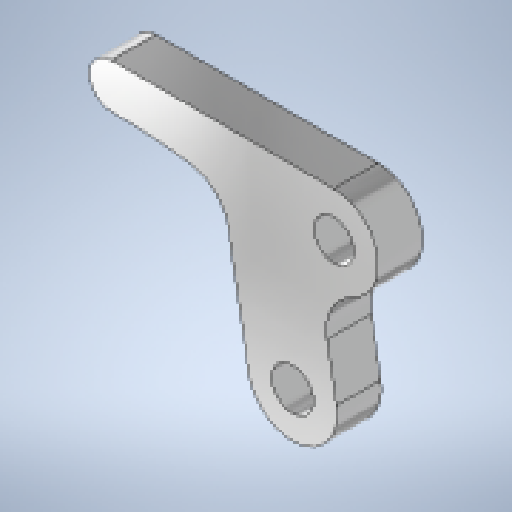
# Autodesk Inventor part: Lever
Saved by Autodesk Inventor 2023.4 (Build 274418000, 418)
## iProperties
Created: 2024-02-17
Part Number: Lever
Material: Aluminum 6061
Document SubType Name: Modeling
Designer: Nathan Cai
Density: 2.7 g/cm^3
Appearance: Aluminum - Flat
Author: Nathan Cai
Autodesk Inventor part; units mm, degrees
ref_plane "YZ Plane" through (0, 0, 0) normal (1, 0, 0) x (0, 1, 0)
ref_plane "XZ Plane" through (0, 0, 0) normal (0, 1, 0) x (-1, 0, 0)
ref_plane "XY Plane" through (0, 0, 0) normal (0, 0, 1) x (1, 0, 0)
sketch "Sketch1" plane through (0, 0, 0) normal (0, 0, 1) x (1, 0, 0)
  circle A0 centre (0, 0) radius 1.4224
  circle A1 centre (0, 0) radius 3.175
  line L0 (0, 0) -> (-19.05, 0) construction
  circle A2 centre (-2.9467, -10.7147) radius 3.175
  circle A3 centre (-2.9467, -10.7147) radius 5 construction
  circle A4 centre (-2.9467, -10.7147) radius 1.5
  line L1 (0, 0) -> (-2.9467, -10.7147) construction
  line L2 (-2.9467, -10.7147) -> (-4.393, -10.3169) construction
  line L3 (0, 0) -> (-2.9467, -10.7147) construction
  arc A5 (-6.0135, -9.8929) -> (0.1201, -11.5364) centre (-2.9467, -10.7147) ccw
  arc A6 (-1.0297, -3.0034) -> (-19.05, 0) centre (-19.05, -55.5625) ccw
  arc A7 (-19.05, 3.175) -> (-19.05, 0) centre (-19.05, 1.5875) ccw
  line L4 (-19.05, 3.175) -> (0, 3.175)
  line L5 (-2.9467, -10.7147) -> (-4.836, 0) construction
  line L6 (0.1801, -10.1634) -> (-1.7092, 0.5513)
  line L7 (-7.9627, -0.5513) -> (-6.0734, -11.266)
  arc A8 (-6.0734, -11.266) -> (0.1801, -10.1634) centre (-2.9467, -10.7147) ccw
  arc A9 (-1.7092, 0.5513) -> (-7.9627, -0.5513) centre (-4.836, 0) ccw
  circle A10 centre (6.7469, -0.7937) radius 3.175
  circle A11 centre (6.7469, -0.7937) radius 1.5
  line L8 (7.1178, 2.3595) -> (0.371, 3.1533)
  arc A12 (4.769, -3.2774) -> (-0.4834, -6.4004) centre (2.7339, -5.8331) ccw
  circle A13 centre (6.7469, -0.7937) radius 5 construction
  point P0 (0.1201, -11.5364)
  point P1 (0, 3.175)
  point P2 (-7.8592, -1.1386)
  point P3 (-6.0734, -11.266)
  point P4 (0.1801, -10.1634)
  point P5 (-1.0859, -2.9835)
  point P6 (-2.418, 2.0577)
  point P7 (0.6312, -3.1116)
  point P8 (1.3474, -2.8749)
  point P9 (-1.4243, -1.0642)
  point P10 (-1.7024, 0.5129)
  point P11 (0.1801, -10.1634)
  dimension "d24" = 3
  dimension "d0" = 2.8448
  dimension "d1" = 6.35
  dimension "d9" = 19.05
  dimension "d22" = 6.35
  dimension "d23" = 10
  dimension "d26" = 11.1125
  dimension "d29" = 3.175
  dimension "d30" = 6.35
  dimension "d31" = 6.35
  dimension "d32" = 3
  dimension "d36" = 10
  dimension "d37" = 100
  dimension "d38" = 4.7625
  dimension "d39" = 6.7469
  dimension "d40" = 0.7937
  constraints: 22 end point, 17 point on circle, 14 tangent, 13 centre point, 6 coincident, 2 point on line, 1 concentric, 1 horizontal, 1 parallel, 1 perpendicular, 3 other
  measures "d0" diameter of A0
  measures "d1" diameter of A1
  measures "d9" distance of L0.start L0.end
  measures "d22" diameter of A2
  measures "d23" diameter of A3
  measures "d26" distance from line of point (0, 0) L2
  measures "d29" diameter of A7
  measures "d30" diameter of A9
  measures "d31" diameter of A10
  measures "d32" diameter of A11
  measures "d36" diameter of A13
  measures "d37" angle of L0 L5
  measures "d38" distance from line of A0.centre L5
  measures "d39" horizontal distance of A0.centre A11.centre
  measures "d40" vertical distance of A0.centre A11.centre
extrude "Extrusion1" add sketch "Sketch1" along normal blind 3.175 contours A1 L6 A9 | A12 L6 A1 | A1 A9 L4 | L6 A2 L7 A6 | A9 L6 A1 | A1 A6 L7 A9 | A9 L7 A6 A7 L4 | A2
fillet "Fillet1" radius 3.175 1 edges at (-7.8592, -1.1386, 1.5875)
sketch "Sketch2" plane through (0, 0, 3.175) normal (0, 0, 1) x (1, 0, 0)
  circle A0 centre (-2.9467, -10.7147) radius 1.5 projected
  circle A1 centre (-2.9467, -10.7147) radius 5.5
  line L0 (0, 3.175) -> (-19.05, 3.175) projected
  arc A2 (-19.05, 3.175) -> (-19.05, 0) centre (-19.05, 1.5875) ccw projected
  arc A3 (-10.0913, -0.727) -> (-19.05, 0) centre (-19.05, -55.5625) ccw projected
  arc A4 (-7.4765, -3.3091) -> (-10.0913, -0.727) centre (-10.6032, -3.8604) ccw projected
  line L1 (-7.4765, -3.3091) -> (-6.0734, -11.266) projected
  arc A5 (-6.0734, -11.266) -> (0.1801, -10.1634) centre (-2.9467, -10.7147) ccw projected
  line L2 (0.1801, -10.1634) -> (-0.4834, -6.4004) projected
  arc A6 (1.3474, -2.8749) -> (-0.4834, -6.4004) centre (2.7339, -5.8331) ccw projected
  arc A7 (1.3474, -2.8749) -> (0, 3.175) centre (0, 0) ccw projected
  circle A8 centre (0, 0) radius 1.4224 projected
  circle A9 centre (-2.9467, -10.7147) radius 1.5 projected
  arc A10 (-7.4765, -3.3091) -> (-10.0913, -0.727) centre (-10.6032, -3.8604) ccw projected
  line L3 (0, 3.175) -> (-19.05, 3.175) projected
  arc A11 (-7.4765, -3.3091) -> (-5.6965, 3.175) centre (-18.3965, 3.175) ccw
  point P0 (-6.8533, -6.8432)
  point P1 (-0.5325, -5.7729)
  point P2 (-5.6965, 3.175)
  dimension "d41" = 11
  dimension "d42" = 12.7
  constraints: 2 centre point, 2 point on circle, 1 coincident, 1 line through centre, 1 point on line
  measures "d41" diameter of A1
  measures "d42" radius of A11
extrude "Extrusion2" add sketch "Sketch2" along normal blind 0.7937 contours A1 L1 A11 L0 A7 A6 | A4 A3 A2 L0 A11
extrude "Extrusion3" add sketch "Sketch2" along normal blind 3.175 contours A1 L1 A11 L0 A7 A6
fillet "Fillet2" radius 1.5875 4 edges at (-6.8533, -6.8432, 4.7625) (-0.5325, -5.7729, 4.7625) (-7.4765, -3.3091, 5.1594) (-5.6965, 3.175, 5.1594)
body "Solid1"
